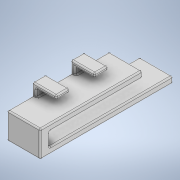
# Autodesk Inventor part: Eyeglasses Side Shields Clip - R
Saved by Autodesk Inventor 2020 (Build 240168000, 168)
## iProperties
Created: 2020-01-16
Part Number: Eyeglasses Side Shields Clip - R
Material: Generic
Document SubType Name: Modeling
Designer: maple
Density: 1 g/cm^3
Appearance: Default
Author: maple
Autodesk Inventor part; units mm, degrees
ref_plane "YZ Plane" through (0, 0, 0) normal (1, 0, 0) x (0, 1, 0)
ref_plane "XZ Plane" through (0, 0, 0) normal (0, 1, 0) x (-1, 0, 0)
ref_plane "XY Plane" through (0, 0, 0) normal (0, 0, 1) x (1, 0, 0)
sketch "Sketch1" plane through (0, 0, 0) normal (0, 1, 0) x (-1, 0, 0)
  line L0 (0, 0) -> (-6.35, 0)
  line L1 (-6.35, 0) -> (-6.35, -25.4)
  line L2 (-6.35, -25.4) -> (0, -25.4)
  line L3 (0, -25.4) -> (0, 0)
  dimension "d0" = 6.35
  dimension "d1" = 25.4
  constraints: 8 end point, 2 parallel, 1 horizontal, 1 perpendicular
  measures "d0" distance of L2.end L1.end
  measures "d1" distance of L1.end L0.end
extrude "Extrusion1" add sketch "Sketch1" along normal blind 1.27
sketch "Sketch2" plane through (0, 1.27, 0) normal (0, 1, 0) x (1, 0, 0)
  line L0 (6.35, 0) -> (6.35, 25.4) projected
  line L1 (0, 0) -> (6.35, 0)
  line L2 (6.35, 0) -> (6.35, 1.7666)
  line L3 (6.35, 1.7666) -> (0, 1.7666)
  line L4 (0, 1.7666) -> (0, 0)
  constraints: 8 end point, 2 parallel, 1 horizontal, 1 perpendicular, 1 point on line
extrude "Extrusion2" add sketch "Sketch2" along normal blind 3.81
sketch "Sketch4" plane through (6.35, 1.27, -1.7666) normal (0, 0, -1) x (-1, 0, 0)
  line L0 (6.35, 3.81) -> (0, 3.81) projected
  line L1 (6.35, -1.27) -> (6.35, 3.81) projected
  line L2 (0, 3.81) -> (6.35, 3.81)
  line L3 (6.35, 3.81) -> (6.35, 2.5394)
  line L4 (6.35, 2.5394) -> (0, 2.5394)
  line L5 (0, 2.5394) -> (0, 3.81)
  constraints: 8 end point, 2 parallel, 1 horizontal, 1 perpendicular, 1 point on line
extrude "Extrusion3" add sketch "Sketch4" along normal blind 17.78
sketch "Sketch5" plane through (0, 5.08, 0) normal (0, 1, 0) x (1, 0, 0)
  line L0 (0, 0) -> (0, 4.826)
  line L1 (0, 1.7666) -> (0, 19.5466) projected
  line L2 (0, 4.826) -> (0.762, 4.826)
  line L3 (0.762, 4.826) -> (0.762, 7.366)
  line L4 (0.762, 7.366) -> (0, 7.366)
  line L5 (0, 7.366) -> (0, 4.826)
  line L6 (0, 7.366) -> (0, 12.192)
  line L7 (0, 12.192) -> (0.762, 12.192)
  line L8 (0.762, 12.192) -> (0.762, 14.732)
  line L9 (0.762, 14.732) -> (0, 14.732)
  line L10 (0, 14.732) -> (0, 12.192)
  dimension "d8" = 4.826
  dimension "d9" = 0.762
  dimension "d10" = 2.54
  dimension "d11" = 4.826
  dimension "d12" = 0.762
  dimension "d13" = 2.54
  constraints: 20 end point, 4 parallel, 2 horizontal, 2 perpendicular, 2 point on line
  measures "d8" distance of L0.start L0.end
  measures "d9" distance of L4.end L3.end
  measures "d10" distance of L3.end L2.end
  measures "d11" distance of L4.end L6.end
  measures "d12" distance of L9.end L8.end
  measures "d13" distance of L8.end L7.end
extrude "Extrusion4" add sketch "Sketch5" along normal blind 2.286
sketch "Sketch6" plane through (0.762, 5.08, -4.826) normal (1, 0, 0) x (0, 0, -1)
  line L0 (2.54, 0) -> (2.54, 2.286) projected
  line L1 (0, 2.286) -> (2.54, 2.286)
  line L2 (2.54, 2.286) -> (2.54, 1.524)
  line L3 (2.54, 1.524) -> (0, 1.524)
  line L4 (0, 1.524) -> (0, 2.286)
  line L5 (7.366, 0) -> (7.366, 2.286) projected
  line L6 (9.906, 0) -> (9.906, 2.286) projected
  line L7 (7.366, 2.286) -> (9.906, 2.286)
  line L8 (9.906, 2.286) -> (9.906, 1.524)
  line L9 (9.906, 1.524) -> (7.366, 1.524)
  line L10 (7.366, 1.524) -> (7.366, 2.286)
  point P0 (-4.826, -5.08)
  point P1 (7.366, 1.524)
  dimension "d16" = 0.762
  dimension "d17" = 0.762
  constraints: 16 end point, 4 parallel, 2 horizontal, 2 perpendicular, 2 point on line
  measures "d16" distance of L1.end L2.end
  measures "d17" distance of L7.end L8.end
extrude "Extrusion5" add sketch "Sketch6" along normal blind 3.81
fillet "Fillet1" radius 0.254 55 edges at (0, 5.08, -9.779) (0, 5.08, -17.1393) (0, 5.08, -2.413) (3.175, 5.08, 0) (0, 7.366, -13.462) (0, 6.223, -14.732) (0, 6.223, -12.192) (2.286, 7.366, -12.192) (2.286, 7.366, -14.732) (0, 6.223, -7.366) (0, 6.223, -4.826) (0, 7.366, -6.096) (4.572, 7.366, -13.462) (4.572, 7.366, -6.096) (2.286, 7.366, -4.826) (2.286, 7.366, -7.366) (4.572, 6.604, -13.462) (0.762, 5.842, -14.732) (0.762, 5.842, -12.192) (2.667, 6.604, -12.192) (4.572, 6.985, -12.192) (4.572, 6.985, -14.732) (4.572, 6.985, -7.366) (4.572, 6.985, -4.826) (4.572, 6.604, -6.096) (0.762, 5.842, -4.826) (0.762, 5.842, -7.366) (2.667, 6.604, -14.732) (0, 3.8094, -10.6566) (0, 2.5397, -1.7666) (0, 2.54, 0) (0, 0, -12.7) (0, 1.27, -13.5833) (6.35, 0, -12.7) (6.35, 1.27, -13.5833) (3.175, 1.27, -25.4) (3.175, 0, -25.4) (6.35, 0.635, -25.4) (0, 0.635, -25.4) (0, 4.4447, -19.5466) (3.175, 3.8094, -19.5466) (3.175, 5.08, -19.5466) (6.35, 5.08, -9.7733) (3.175, 0, 0) (6.35, 2.54, 0) (6.35, 2.5397, -1.7666) (6.35, 3.8094, -10.6566) (6.35, 4.4447, -19.5466) (2.667, 6.604, -4.826) (2.667, 6.604, -7.366) (0.762, 6.604, -6.096) (3.175, 3.8094, -1.7666) (3.175, 1.27, -1.7666) (0.762, 5.08, -13.462) (0.762, 5.08, -6.096)
body "Solid1"
